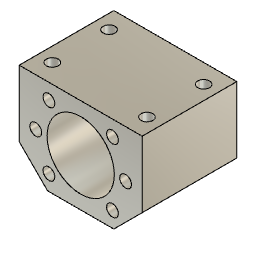
Ballnut Housing 28mm (Autodesk Fusion 360 design; units mm, degrees)
Autodesk Fusion 360 part; units mm, degrees
sketch "Housing Front" plane through (0, 0, 0) normal (0, 1, 0) x (1, 0, 0)
  circle A0 centre (0, 0) radius 14.2
  line L0 (-26, -20) -> (26, -20)
  line L1 (26, -20) -> (26, 8)
  line L2 (26, 8) -> (14, 20)
  line L3 (14, 20) -> (-14, 20)
  line L4 (-14, 20) -> (-26, 8)
  line L5 (-26, 8) -> (-26, -20)
  circle A1 centre (-19, 0) radius 2.5
  circle A2 centre (-19, 0) radius 2.5
  circle A3 centre (-13.435, 13.435) radius 2.5
  circle A4 centre (-13.435, -13.435) radius 2.5
  circle A5 centre (13.435, 13.435) radius 2.5
  circle A6 centre (19, 0) radius 2.5
  circle A7 centre (13.435, -13.435) radius 2.5
  dimension "d1" = 28.4
  dimension "d2" = 52
  dimension "d3" = 26
  dimension "d4" = 20
  dimension "d5" = 40
  dimension "d6" = 12
  dimension "d7" = 12
  dimension "d8" = 5
  dimension "d9" = 19
  dimension "d10" = 5
  dimension "d11" = 5
  dimension "d12" = 5
  dimension "d13" = 5
  dimension "d14" = 5
  dimension "d15" = 5
  constraint coincident A0.centre origin
  constraint horizontal L0
  constraint perpendicular L0 L1
  constraint perpendicular L1 L3
  constraint perpendicular L0 L5
  constraint equal L1 L5
  constraint equal L2 L4
  measures "d1" diameter of A0
  measures "d2" distance of L1 L5
  measures "d3" distance of A0.centre L5
  measures "d4" distance of A0.centre L0
  measures "d5" distance of L0 L3
  measures "d6" vertical distance of L3.end L4.end
  measures "d7" horizontal distance of L3.end L4.end
  measures "d8" diameter of A1
  measures "d9" distance of A0.centre A1.centre
  measures "d10" diameter of A2
  measures "d11" diameter of A3
  measures "d12" diameter of A4
  measures "d13" diameter of A6
  measures "d14" diameter of A7
  measures "d15" diameter of A5
  measures "d25" diameter of A0.centre
  measures "d27" diameter of A0.centre
extrude "Extrude1" add sketch "Housing Front" along normal blind 40 makes body 1
extrude "Extrude2" add sketch "Housing Front" along normal blind 28 contours A1 A2 | A3 | A4 | A5 | A6 | A7 bodies 1
sketch "Housing Top" plane through (0, 0, 20) normal (0, 0, 1) x (-1, 0, 0)
  line L0 (26, 0) -> (-26, 0)
  line L1 (-26, 0) -> (-26, -40)
  line L2 (-26, -40) -> (26, -40)
  line L3 (26, -40) -> (26, 0)
  line L4 (20, -8) -> (-20, -8) construction
  line L5 (-20, -8) -> (-20, -32) construction
  line L6 (-20, -32) -> (20, -32) construction
  line L7 (20, -32) -> (20, -8) construction
  circle A0 centre (20, -32) radius 2.5
  circle A1 centre (-20, -32) radius 2.5
  circle A2 centre (20, -8) radius 2.5
  circle A3 centre (-20, -8) radius 2.5
  dimension "d20" = 40
  dimension "d21" = 24
  dimension "d22" = 8
  dimension "d23" = 6
  dimension "d24" = 5
  dimension "d25" = 5
  dimension "d26" = 5
  dimension "d27" = 5
  constraint perpendicular L1 L4
  constraint perpendicular L4 L5
  constraint perpendicular L5 L6
  constraint perpendicular L4 L7
  constraint coincident L6.end L7.start
  constraint coincident L5.end L6.start
  constraint coincident L4.start L7.end
  constraint coincident L4.end L5.start
  measures "d20" distance of L5 L7
  measures "d21" distance of L4 L6
  measures "d22" distance of L2 L6
  measures "d23" distance of L1 L5
  measures "d24" diameter of A0
  measures "d25" diameter of A1
  measures "d26" diameter of A2
  measures "d27" diameter of A3
extrude "Extrude3" cut sketch "Housing Top" against normal blind 12 contours A0 | A1 | A2 | A3 bodies 1
move_body "Move1" bodies 1 to x (-1, 0, 0) y (0, -1, 0) z (0, 0, 1) at (0, 0, 0)
move_body "Move2" bodies 1 to x (1, 0, 0) y (0, 1, 0) z (0, 0, 1) at (0, 20, 0)
copy_body "Body->Comp1" bodies 1 removing the originals makes body 2 in component "Ballnut Housing 28mm"
component "Ballnut Housing 28mm" placed x (1, 0, 0) y (0, 1, 0) z (0, 0, 1) at (0, 0, 0)
named bodies: "Ballnut Housing 28mm"
